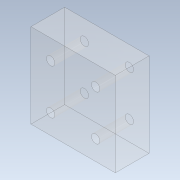
# Autodesk Inventor part: Part15
Saved by Autodesk Inventor 2021.1 (Build 251245010, 245A)
## iProperties
Created: 2023-10-18
Part Number: Part15
Material: PMMA Plastic
Document SubType Name: Modeling
Designer: Lenovo
Density: 1.188 g/cm^3
Appearance: Polycarbonate - Clear
Author: Lenovo
Autodesk Inventor part; units mm, degrees
ref_plane "YZ Plane" through (0, 0, 0) normal (1, 0, 0) x (0, 1, 0)
ref_plane "XZ Plane" through (0, 0, 0) normal (0, 1, 0) x (-1, 0, 0)
ref_plane "XY Plane" through (0, 0, 0) normal (0, 0, 1) x (1, 0, 0)
ref_plane "Work Plane1" through (0, 0, 0) normal (0, 0, 1) x (1, 0, 0)
sketch "Sketch1" plane through (0, 0, 0) normal (0, 0, 1) x (1, 0, 0)
  circle A0 centre (259.2722, 267.3165) radius 3
  circle A1 centre (259.2722, 267.3165) radius 3
  line L0 (273.2722, 221.3165) -> (213.2722, 221.3165)
  line L1 (213.2722, 221.3165) -> (213.2722, 281.3165)
  line L2 (213.2722, 281.3165) -> (273.2722, 281.3165)
  line L3 (273.2722, 281.3165) -> (273.2722, 221.3165)
  line L4 (273.2722, 221.3165) -> (213.2722, 281.3165) construction
  line L5 (213.2722, 221.3165) -> (273.2722, 281.3165) construction
  circle A2 centre (227.2722, 267.3165) radius 3
  circle A3 centre (227.2722, 235.3165) radius 3
  circle A4 centre (259.2722, 235.3165) radius 3
  line L6 (227.2722, 235.3165) -> (259.2722, 235.3165)
  line L7 (227.2722, 267.3165) -> (227.2722, 235.3165)
  line L8 (259.2722, 267.3165) -> (259.2722, 235.3165)
  line L9 (259.2722, 267.3165) -> (227.2722, 267.3165)
  point P0 (0, 0)
  dimension "d0" = 60
  dimension "d1" = 60
  dimension "d4" = 6
  dimension "d5" = 6
  dimension "d6" = 6
  dimension "d11" = 6
  dimension "d12" = 14
  dimension "d14" = 14
  dimension "d15" = 32
  constraints: 20 end point, 5 centre point, 3 perpendicular, 2 horizontal, 2 parallel, 1 point on line, 1 vertical
  measures "d0" distance of L1.end L2.end
  measures "d1" distance of L0.end L1.end
  measures "d4" diameter of A2
  measures "d5" diameter of A3
  measures "d6" diameter of A4
  measures "d11" diameter of A0
  measures "d12" distance between parallel lines of L2 L9
  measures "d14" distance between parallel lines of L3 L8
  measures "d15" distance of L8.start L7.start
extrude "Extrusion1" add sketch "Sketch1" along normal blind 24 contours A0 L8 A4 L6 A3 L7 A2 L9 | L0 L1 L2 L3
equation "\"d4\" = d5"
equation "\"d6\" = d5"
equation "\"d11\" = d5"
body "Solid1"
